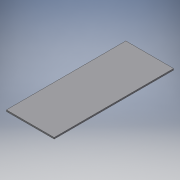
# Autodesk Inventor part: ChapaFrontalCabecaAquevimento
Saved by Autodesk Inventor 2018 (Build 220112000, 112)
## iProperties
Created: 2018-09-22
Part Number: ChapaFrontalCabecaAquevimento
Material: Genérico
Document SubType Name: Chapa de metal
Designer: Usuario
Density: 1 g/cm^3
Sheet Metal Rule: Padrão_mm
Appearance: Padrão
Author: Usuario
Autodesk Inventor part; units mm, degrees
ref_plane "YZ Plane" through (0, 0, 0) normal (1, 0, 0) x (0, 1, 0)
ref_plane "XZ Plane" through (0, 0, 0) normal (0, 1, 0) x (-1, 0, 0)
ref_plane "XY Plane" through (0, 0, 0) normal (0, 0, 1) x (1, 0, 0)
sketch "Esboço1" plane through (0, 0, 0) normal (0, 0, 1) x (1, 0, 0)
  line L0 (-75, 50) -> (75, 50)
  line L1 (75, 50) -> (75, -50)
  line L2 (75, -50) -> (-75, -50)
  line L3 (-75, -50) -> (-75, 50)
  line L4 (-75, 50) -> (75, -50) construction
  line L5 (75, 50) -> (-75, -50) construction
  point P0 (0, 0)
  dimension "d0" = 150
  dimension "d1" = 100
  measures "d0" distance of L0.start L0.end
  measures "d1" distance of L0.end L1.end
extrude "Placa1" add sketch "Esboço1" along normal blind 3
equation "\"d2\" = Espessura"
equation "\"Raio_vergadura\" = Espessura"
equation "\"Largura_alívio_de_vergadura\" = Espessura"
equation "\"Profundidade_alívio_de_vergadura\" = 0.5 * Espessura"
equation "\"Tamanho_alívio_de_dobra\" = 4 * Espessura"
equation "\"Remanescente_mínimo\" = 2 * Espessura"
equation "\"Raiodetransição\" = Raio_vergadura"
equation "\"Tamanho_de_raio_de_Jacobi\" = Raio_vergadura"
equation "\"TamanhoFolga\" = Espessura"
equation "\"Espessura\" = 3"
